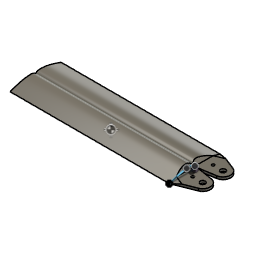
Rotor v2 v8 (Autodesk Fusion 360 archive; units mm, degrees)
design "rotor blade"
Autodesk Fusion 360 part; units mm, degrees
sketch "Sketch1" plane through (0, 0, 0) normal (1, 0, 0) x (0, 0, -1)
  line L0 (0, 0) -> (-20, 0)
  spline S0 degree 5 poles (-2.5, 0) (-2.2697, 0) (-1.8074, 0.0307) (-1.1086, 0.1684) (-0.2592, 0.5655) (0.265, 1.4519) (-0.0728, 2.5892) (-1.1618, 3.3882) (-2.7222, 3.7471) (-4.4389, 3.7644) (-6.0558, 3.6395) (-7.5324, 3.4826) (-9.0781, 3.222) (-10.7741, 2.8475) (-12.6889, 2.3422) (-14.8487, 1.7043) (-16.7818, 1.0877) (-18.3465, 0.5665) (-19.4404, 0.1932) (-20, 0) knots 0 0 0 0 0 0 0.066667 0.133333 0.2 0.266667 0.333333 0.4 0.466667 0.533333 0.6 0.666667 0.733333 0.8 0.866667 0.933333 1 1 1 1 1 1
  line L1 (-5, 0) -> (0, 0)
  line L2 (-4.5261, 3.7824) -> (-8.2569, 3.4076)
  line L3 (0.4463, 0.5042) -> (-0.4463, 3.4958)
  point P0 (-2.5, 0)
  point P1 (0, 2)
  point P2 (0, 2)
  point P3 (-6.3915, 3.595)
  dimension "d1" = 20
  dimension "d2" = 2.5
  dimension "d3" = 2
  constraint coincident L0.start L1.end
  constraint horizontal L0
  constraint coincident L0 P0
  constraint coincident P0 S0.start
  constraint coincident P2 P1
  constraint midpoint P0 L1
  constraint coincident L0 L1.start
  constraint midpoint P3 L2
  constraint midpoint P2 L3
  measures "d1" distance of L0.start L0.end
  measures "d2" distance of L0.start S0.start
  measures "d3" distance of L0.start P2
sketch "Sketch2" plane through (0, 0, 0) normal (0, 1, 0) x (1, 0, 0)
  line L0 (0, 0) -> (0, -20)
  line L1 (0, -12) -> (20.3, -12) construction
  line L2 (20.3, -8) -> (20.3, -4) construction
  line L3 (20.3, -4) -> (0, -4) construction
  line L4 (0, -4) -> (0, -12)
  circle A0 centre (14.2, -8) radius 6.1 construction
  line L5 (0, -8) -> (20.3, -8) construction
  circle A1 centre (14.2, -8) radius 2
  circle A2 centre (6.35, -8) radius 1.05
  line L6 (0, -20) -> (16.384, -13.5347)
  line L7 (20.3, -12) -> (20.3, -8) construction
  arc A3 (15.0265, -2.1077) -> (9.7952, -4) centre (14.2, -8) ccw construction
  arc A4 (9.7952, -4) -> (9.7952, -12) centre (14.2, -8) ccw construction
  arc A5 (16.384, -13.5347) -> (15.0265, -2.1077) centre (14.2, -8) ccw
  arc A6 (9.7952, -12) -> (16.384, -13.5347) centre (14.2, -8) ccw construction
  line L8 (0, 0) -> (0, 0.3)
  line L9 (0, 0.3) -> (15.0265, -2.1077)
  point P0 (0, -10)
  point P1 (0, -10)
  point P2 (0, -6.3915)
  dimension "d7" = 20.3
  dimension "d8" = 8
  dimension "d9" = 20
  dimension "d10" = 12.2
  dimension "d11" = 4
  dimension "d12" = 2.1
  dimension "d13" = 7.85
  dimension "d25" = 4
  dimension "d26" = 4
  dimension "d27" = 5.95
  dimension "d28" = 0.3
  constraint coincident L0.start L8.start
  constraint vertical L0
  constraint horizontal L1
  constraint vertical L2
  constraint horizontal L3
  constraint vertical L4
  constraint coincident P1 P0
  constraint coincident A0.centre L5
  constraint tangent L2 A0
  constraint concentric A0 A1
  constraint coincident L5 A2.centre
  constraint coincident L6.end A4
  constraint tangent L6 A4
  constraint vertical L7
  constraint concentric A0 A4
  constraint coincident L3 A3.end
  constraint concentric A3 A4
  constraint coincident L1 A4.end
  constraint concentric A4 A5
  constraint concentric A4 A6
  constraint midpoint L4 L5.start
  constraint coincident L4 P2
  constraint parallel L0 L8
  measures "d7" distance of L1.start L1.end
  measures "d8" distance of L1.end L2.end
  measures "d9" distance of L0.start L0.end
  measures "d10" diameter of A0
  measures "d11" diameter of A1
  measures "d12" diameter of A2
  measures "d13" distance of A0.centre A2.centre
  measures "d25" distance of L0.start L3
  measures "d26" distance of L2.end L2.start
  measures "d27" radius of A5
  measures "d28" distance of L0.start L8.end
extrude "Extrude2" add sketch "Sketch2" along normal blind 1.85 makes body 1
extrude "Extrude3" cut sketch "Sketch1" along normal blind 21 draft 7 keep common part bodies 1
extrude "Extrude4" add sketch "Sketch1" against normal blind 125 bodies 1
draft "Draft1" angle 60 neutral plane through (0, 1.85, 0) pull (0, 1, 0) 1 faces at (0, 2.2412, 8.0734) on bodies 1
mirror "Mirror1" about plane through (0, 0, 0) normal (0, 0, 1) of bodies 1 makes body 2
equation "d15 = 2.45 mm - 0.6 mm"
equation "d27 = 6.1 mm - 0.15 mm"

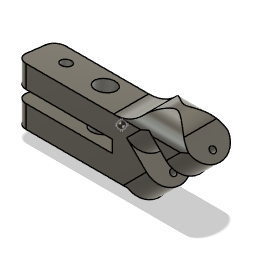
design "Blade Holder v2"
Autodesk Fusion 360 part; units mm, degrees
sketch "Sketch4" plane through (0, 0, 0) normal (0, 0, 1) x (1, 0, 0)
  line L0 (5.16, -2.9698) -> (8.6955, 0.5657) construction
  line L1 (8.6955, 0.5657) -> (5.16, 4.1012) construction
  line L2 (5.16, 4.1012) -> (1.6244, 0.5657) construction
  line L3 (1.6244, 0.5657) -> (5.16, -2.9698) construction
  line L4 (0, 0) -> (9.9337, 0) construction
  line L5 (5.16, -3.3941) -> (9.1198, 0.5657) construction
  line L6 (9.1198, 0.5657) -> (5.16, 4.5255)
  line L7 (5.16, 4.5255) -> (1.2002, 0.5657)
  line L8 (1.2002, 0.5657) -> (5.16, -3.3941)
  line L9 (9.1198, 0.5657) -> (13.0796, 4.5255)
  line L10 (13.0796, 4.5255) -> (9.1183, 8.4868)
  line L11 (5.16, -3.3941) -> (0.9173, -7.6368)
  line L12 (0.9173, -7.6368) -> (-1.4944, -5.225)
  arc A0 (1.2032, 8.4883) -> (9.1198, 0.5657) centre (5.16, 4.5255) ccw construction
  arc A1 (9.1183, 8.4868) -> (1.2032, 8.4883) centre (5.16, 4.5255) ccw
  arc A2 (9.1198, 0.5657) -> (9.1183, 8.4868) centre (5.16, 4.5255) ccw construction
  line L13 (9.1183, 8.4868) -> (5.16, 12.4451) construction
  line L14 (-23.4998, -0.925) -> (-4.7998, -0.925) construction
  line L15 (-4.7998, -0.925) -> (-4.7998, 0.925) construction
  line L16 (-4.7998, 0.925) -> (-23.4998, 0.925) construction
  line L17 (-23.4998, 0.925) -> (-23.4998, -0.925) construction
  line L18 (-23.7998, -1.225) -> (-4.4998, -1.225)
  line L19 (-4.4998, -1.225) -> (-4.4998, 1.225)
  line L20 (-4.4998, 1.225) -> (-23.7998, 1.225)
  line L21 (-23.7998, 1.225) -> (-23.7998, -1.225) construction
  line L22 (-23.7998, 1.225) -> (-23.7998, 5.225)
  line L23 (-23.7998, 5.225) -> (-2.0601, 5.225)
  line L24 (-23.7998, -1.225) -> (-23.7998, -5.225)
  line L25 (-23.7998, -5.225) -> (-1.4944, -5.225)
  line L26 (-4.7998, -1.9196) -> (-7.0023, 0.2828) construction
  line L27 (-4.4998, -2.2196) -> (-4.7998, -1.9196) construction
  line L28 (-1.4944, -5.225) -> (-4.4998, -2.2196) construction
  line L29 (-1.4944, 5.225) -> (-1.4944, -5.225) construction
  line L30 (7.4934, 1.7678) -> (3.9579, -1.7678) construction
  line L31 (-7.0023, 0.2828) -> (-4.7998, 2.4853) construction
  line L32 (-2.0601, 5.225) -> (1.2032, 8.4883)
  line L33 (-4.7998, 2.4853) -> (-2.0601, 5.225) construction
  line L34 (1.2032, 8.4883) -> (5.16, 12.4451) construction
  line L35 (-2.0601, 5.225) -> (-1.4944, 5.225) construction
  line L36 (-4.4998, 1.225) -> (-4.4998, 5.225)
  line L37 (-4.4998, -1.225) -> (-4.4998, -5.225)
  point P0 (-4.7998, 0)
  point P1 (5.7257, 0)
  point P2 (-17.3998, 1.225)
  point P3 (-19.4998, 1.225)
  dimension "d55" = 45
  dimension "d57" = 5.6
  dimension "d58" = 11.2
  dimension "d59" = 5.6
  dimension "d60" = 6
  dimension "d61" = 11.2
  dimension "d63" = 18.7
  dimension "d66" = 4
  dimension "d67" = 4
  dimension "d84" = 5
  dimension "d85" = 2
  dimension "d86" = 5.7
  dimension "d91" = 12.9
  dimension "d92" = 2.1
  dimension "d93" = 4.3
  dimension "d94" = 45
  dimension "d99" = 2.45
  dimension "d116" = 19.3
  constraint horizontal L4
  constraint perpendicular L0 L3
  constraint perpendicular L0 L1
  constraint perpendicular L1 L2
  constraint perpendicular L6 L9
  constraint perpendicular L9 L10
  constraint perpendicular L8 L11
  constraint perpendicular L11 L12
  constraint coincident L6.end L7.start
  constraint tangent L10 A0
  constraint concentric A0 A1
  constraint concentric A0 A2
  constraint perpendicular L9 L13
  constraint horizontal L14
  constraint vertical L15
  constraint horizontal L16
  constraint vertical L17
  constraint midpoint L15 P0
  constraint coincident L4 P0
  constraint perpendicular L20 L22
  constraint perpendicular L22 L23
  constraint perpendicular L18 L24
  constraint perpendicular L24 L25
  constraint coincident L15 L26.start
  constraint perpendicular L11 L26
  constraint coincident L19 L27.start
  constraint perpendicular L11 L27
  constraint perpendicular L11 L28
  constraint perpendicular L25 L29
  constraint coincident L1 L30.start
  constraint coincident L3 L30.end
  constraint perpendicular L3 L30
  constraint midpoint L30 P1
  constraint coincident L4 P1
  constraint coincident L0.start L3.end
  constraint coincident L2.end L3.start
  constraint coincident L1.end L2.start
  constraint coincident L0.end L1.start
  constraint coincident L15 L31.end
  constraint coincident A1 A0.start
  constraint coincident L20 P2
  constraint coincident L20 P3
  constraint collinear L32 L34
  constraint collinear L31 L32
  constraint coincident A0.start A1.end
  constraint perpendicular L22 L35
  constraint coincident L23 L36.end
  constraint perpendicular L23 L36
  constraint coincident L25 L37.end
  constraint perpendicular L25 L37
  measures "d55" angle of L3 L4
  measures "d57" distance of L5.end L9.end
  measures "d58" distance of L9.end L13.end
  measures "d59" distance of L5.end L6.end
  measures "d60" distance of L5.start L11.end
  measures "d61" distance of L11.end L26.end
  measures "d63" distance of L14.start L14.end
  measures "d66" distance of L20.end L22.end
  measures "d67" distance of L18.start L24.end
  measures "d84" distance of L30.start L30.end
  measures "d85" distance of L5.end L30
  measures "d86" distance of L7.end L19
  measures "d91" distance of L19 P2
  measures "d92" distance of P2 P3
  measures "d93" distance of L20.end P3
  measures "d94" angle of L4 L32
  measures "d99" distance of L18 L20
  measures "d116" distance of L22 L36
extrude "Extrude4" add sketch "Sketch4" along normal mid plane 8 contours L6 L7 L8 L9 L10 L11 L12 A1 L19 L23 L25 L32 L36 L37
sketch "Sketch8" plane through (-4.4998, 0, 0) normal (-1, 0, 0) x (0, 0, 1)
  line L0 (-4, -5.225) -> (4, -5.225)
  line L1 (4, -5.225) -> (4, 5.225)
  line L2 (4, 5.225) -> (-4, 5.225)
  line L3 (-4, 5.225) -> (-4, -5.225)
  line L4 (-0.1493, 1.2159) -> (0.1493, -1.2159)
  line L5 (0, -5.225) -> (0, 5.225) construction
  line L6 (-0.1493, 1.2159) -> (-4, 0.7431)
  line L7 (0.1493, -1.2159) -> (-4, -1.7253)
  line L8 (0.1493, -1.2159) -> (4, -0.7431)
  line L9 (-0.1493, 1.2159) -> (4, 1.7253)
  line L10 (4, 8.4868) -> (4, 10.1255)
  line L11 (-4, 10.1255) -> (-4, 8.4868)
  line L12 (-4, 10.1255) -> (4, 10.1255)
  line L13 (4, 10.1255) -> (4, -7.6368)
  line L14 (4, -7.6368) -> (-4, -7.6368)
  line L15 (-4, -7.6368) -> (-4, 10.1255)
  circle A0 centre (0, 6.2073) radius 4
  line L16 (-4, 5.225) -> (4, 6.2073)
  line L17 (4, -5.225) -> (-4, -6.2073)
  line L18 (4, 6.2073) -> (-4, 6.2073) construction
  point P0 (-4, -7.6368)
  point P1 (4, -7.6368)
  dimension "d117" = 2.45
  dimension "d118" = 7
  constraint midpoint origin L4
  constraint midpoint L0 L5.start
  constraint midpoint L2 L5.end
  constraint coincident L3 L6.end
  constraint perpendicular L4 L6
  constraint coincident L3 L7.end
  constraint perpendicular L4 L7
  constraint coincident L1 L8.end
  constraint perpendicular L4 L8
  constraint coincident L1 L9.end
  constraint perpendicular L4 L9
  constraint horizontal L12
  constraint vertical L13
  constraint horizontal L14
  constraint vertical L15
  constraint coincident P1 L13.end
  constraint coincident L11.start L12.start
  constraint tangent L13 A0
  constraint tangent L15 A0
  constraint coincident L2.end L3.start
  constraint coincident L13 L16.end
  constraint parallel L9 L16
  constraint coincident L0.end L1.start
  constraint coincident L15 L17.end
  constraint parallel L8 L17
  constraint coincident A0 L18.end
  constraint perpendicular L15 L18
  constraint midpoint A0.centre L18
  measures "d117" distance of L4.start L4.end
  measures "d118" angle of L4 L5
extrude "Extrude9" add sketch "Sketch8" along normal blind 19.3 and the other way blind 4 contours L0 L1 L3 L7 L8 L13 L15 | L0 L15 L17 | L1 L2 L3 L6 L9 L13 L15 A0 | L2 A0 L16 | L2 L13 A0 | L2 A0 L16 | L2 A0
fillet "Fillet8" radius 7.5 1 edges at (-1.569, 5.7161, 0)
sketch "Sketch5" plane through (8.8025, 8.8025, 0) normal (0.707107, 0.707107, 0) x (0, 0, -1)
  line L0 (3.3989, 2.7494) -> (-3.6389, 2.7493)
  line L1 (-3.6389, 2.7493) -> (-4, -6.0486)
  line L2 (-4, -6.0486) -> (3.9993, -5.9802)
  line L3 (3.9993, -5.9802) -> (3.3989, 2.7494)
  line L4 (-0.0003, -6.0144) -> (-0.0174, -4.0145) construction
  circle A0 centre (-0.0174, -4.0145) radius 0.6
  point P0 (-4, -6.0486)
  dimension "d76" = 2
  dimension "d77" = 1.2
  constraint midpoint L2 L4.start
  constraint perpendicular L2 L4
  constraint coincident L4.end A0.centre
  measures "d76" distance of L4.start L4.end
  measures "d77" diameter of A0
extrude "Extrude5" cut sketch "Sketch5" against normal blind 22 contours A0
fillet "Fillet9" radius 4 6 edges at (11.0997, 2.5456, 4) (11.0997, 2.5456, -4) (3.0386, -5.5154, -4) (3.0386, -5.5154, 4) (3.1801, 2.5456, 4) (3.1801, 2.5456, -4)
fillet "Fillet12" radius 2 4 edges at (-23.7998, 3.9663, 4) (-23.7998, 2.984, -4) (-23.7998, -3.9663, -4) (-23.7998, -2.984, 4)
ref_plane "WorkPlane1" through (-14.1498, 0.0183, 0.1493) normal (0, -0.992546, 0.121869) x (0, 0.121869, 0.992546)
sketch "Sketch7" plane through (0, 0, 0) normal (0, -0.992546, 0.121869) x (1, 0, 0)
  arc A0 (-23.7998, -3) -> (-22.7998, -4) centre (-22.7998, -3) ccw
  line L0 (-22.7998, -4) -> (-4.4998, -4)
  line L1 (-4.4998, -4) -> (-4.4998, 4)
  line L2 (-4.4998, 4) -> (-22.7998, 4)
  arc A1 (-22.7998, 4) -> (-23.7998, 3) centre (-22.7998, 3) ccw
  line L3 (-23.7998, 3) -> (-23.7998, -3)
  circle A2 centre (-18.4498, 0) radius 1.05
  line L4 (-4.4998, 0) -> (-18.4498, 0)
  circle A3 centre (-10.5998, 0) radius 1.8 construction
  circle A4 centre (-10.5998, 0) radius 2
  circle A5 centre (-10.5998, 0) radius 6.1
  line L5 (-4.4998, -4) -> (-4.2, -4)
  line L6 (-4.2, -4) -> (-4.2, 4)
  line L7 (-4.2, 4) -> (-4.4998, 4)
  line L8 (-4.4998, 4) -> (-4.4998, -4)
  circle A6 centre (-18.4498, 0) radius 1.05
  point P0 (-8.7998, 0)
  dimension "d100" = 4.3
  dimension "d101" = 3.6
  dimension "d102" = 0.2
  dimension "d110" = 19.3
  dimension "d111" = 8
  dimension "d112" = 12.2
  dimension "d113" = 4
  dimension "d114" = 2.1
  dimension "d115" = 7.85
  constraint midpoint L1 L4.start
  constraint coincident A2.centre L4.end
  constraint coincident L4 P0
  constraint coincident L4 A3.centre
  constraint coincident P0 A3
  constraint concentric A3 A5
  constraint coincident L4.start A5
  constraint horizontal L5
  constraint vertical L6
  constraint horizontal L7
  constraint vertical L8
  constraint coincident L0.end L1.start
  constraint concentric A2 A6
  measures "d100" distance of L1 P0
  measures "d101" diameter of A3
  measures "d110" distance of L3 L8
  measures "d111" distance of L0 L2
  measures "d112" diameter of A5
  measures "d113" diameter of A4
  measures "d114" diameter of A2
  measures "d115" distance of A2.centre A3.centre
extrude "Extrude7" cut sketch "Sketch7" along normal mid plane 18 contours L4 A4 | L4 A4 | A2 A6
extrude "Extrude10" cut sketch "Sketch8" against normal blind 20 contours L11 L12 L15 A0 | L10 L12 L13 A0
equation "d91 = 7.9 mm + 5 mm"
equation "d99 = 2.95 mm - 0.5 mm"
equation "d121 = ( 2.45 / 2 ) * 1 mm"
